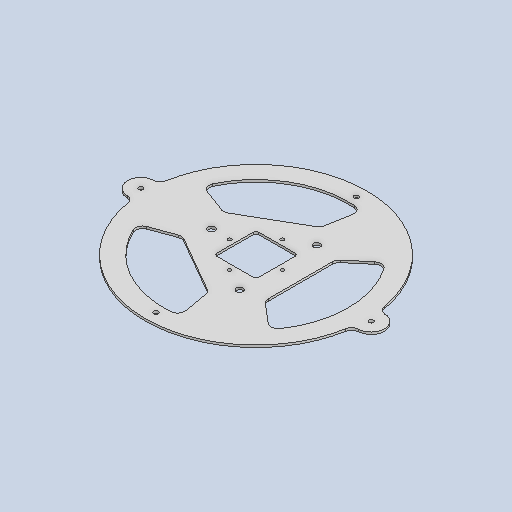
# Autodesk Inventor part: Part1
Saved by Autodesk Inventor 2025.1 (Build 291241020, 241B)
## iProperties
Created: 2024-10-16
Part Number: Part1
Material: Generic
Document SubType Name: Modeling
Designer: jdl5984
Density: 1 g/cm^3
Appearance: Default
Author: jdl5984
Autodesk Inventor part; units mm, degrees
ref_plane "YZ Plane" through (0, 0, 0) normal (1, 0, 0) x (0, 1, 0)
ref_plane "XZ Plane" through (0, 0, 0) normal (0, 1, 0) x (-1, 0, 0)
ref_plane "XY Plane" through (0, 0, 0) normal (0, 0, 1) x (1, 0, 0)
sketch "Sketch1" plane through (0, 0, 0) normal (0, 1, 0) x (-1, 0, 0)
  circle A0 centre (0, 0) radius 158.75
  line L0 (26.05, 30.05) -> (-26.05, 30.05)
  line L1 (-30.05, 26.05) -> (-30.05, -26.05)
  line L2 (-26.05, -30.05) -> (26.05, -30.05)
  line L3 (30.05, -26.05) -> (30.05, 26.05)
  arc A1 (30.05, 26.05) -> (26.05, 30.05) centre (26.05, 26.05) ccw
  arc A2 (26.05, -30.05) -> (30.05, -26.05) centre (26.05, -26.05) ccw
  arc A3 (-30.05, -26.05) -> (-26.05, -30.05) centre (-26.05, -26.05) ccw
  arc A4 (-26.05, 30.05) -> (-30.05, 26.05) centre (-26.05, 26.05) ccw
  circle A5 centre (38, 0) radius 2.5527
  circle A6 centre (0, -38) radius 2.5527
  circle A7 centre (-38, 0) radius 2.5527
  circle A8 centre (0, 38) radius 2.5527
  circle A9 centre (63.9092, 0) radius 4.7625
  circle A10 centre (-31.9546, -55.3454) radius 4.7625
  circle A11 centre (0, 0) radius 63.9092 construction
  circle A12 centre (0, 143.6497) radius 3.2067
  circle A13 centre (0, -143.6497) radius 3.2067
  line L4 (157.6029, 19.05) -> (165.227, 19.05)
  line L5 (165.227, 19.05) -> (165.227, -19.05) construction
  line L6 (165.227, -19.05) -> (157.6029, -19.05)
  line L7 (157.6029, -17.4578) -> (157.6029, 19.05) construction
  arc A14 (165.227, -19.05) -> (165.227, 19.05) centre (165.227, 0) ccw
  circle A15 centre (165.227, 0) radius 3.2067
  line L8 (0, -158.75) -> (0, 158.75) construction
  line L9 (-157.6029, 19.05) -> (-165.227, 19.05)
  line L10 (-165.227, -19.05) -> (-157.6029, -19.05)
  arc A16 (-165.227, 19.05) -> (-165.227, -19.05) centre (-165.227, 0) ccw
  circle A17 centre (-165.227, 0) radius 3.2067
  circle A18 centre (-31.9533, 55.3478) radius 4.7625
  point P0 (30.05, 30.05)
  point P1 (-30.05, 30.05)
  point P2 (30.05, -30.05)
  dimension "d0" = 317.5
  dimension "d1" = 30.05
  dimension "d2" = 60.1
  dimension "d3" = 60.1
  dimension "d4" = 30.05
  dimension "d5" = 4
  dimension "d6" = 4
  dimension "d7" = 5.1054
  dimension "d8" = 5.1054
  dimension "d9" = 5.1054
  dimension "d10" = 5.1054
  dimension "d11" = 76
  dimension "d12" = 38
  dimension "d13" = 76
  dimension "d14" = 38
  dimension "d15" = 9.525
  dimension "d17" = 110.6932
  dimension "d20" = 9.525
  dimension "d24" = 6.4135
  dimension "d25" = 6.4135
  dimension "d26" = 287.2994
  dimension "d27" = 143.6497
  dimension "d30" = 38.1
  dimension "d31" = 6.4135
  dimension "d33" = 330.454
  dimension "d38" = 110.6932
  dimension "d39" = 110.6932
  dimension "d41" = 127.8184
  constraints: 22 end point, 20 point on circle, 19 centre point, 8 tangent, 6 point on line, 6 symmetric about line, 4 coincident, 4 horizontal alignment, 4 parallel, 4 vertical alignment, 3 equal radius, 2 horizontal, 2 perpendicular, 1 midpoint, 1 vertical, 2 other
  measures "d0" diameter of A0
  measures "d1" distance from line of point (0, 0) L3
  measures "d2" distance of point (30.05, 30.05) point (-30.05, 30.05)
  measures "d3" distance of point (30.05, -30.05) point (30.05, 30.05)
  measures "d4" distance from line of point (0, 0) L2
  measures "d5" radius of A1
  measures "d6" radius of A2
  measures "d7" diameter of A5
  measures "d8" diameter of A6
  measures "d9" diameter of A7
  measures "d10" diameter of A8
  measures "d11" distance of A7.centre A5.centre
  measures "d12" distance of point (0, 0) A7.centre
  measures "d13" distance of A8.centre A6.centre
  measures "d14" distance of point (0, 0) A6.centre
  measures "d15" diameter of A9
  measures "d17" distance of A10.centre A9.centre
  measures "d20" diameter of A10
  measures "d24" diameter of A13
  measures "d25" diameter of A12
  measures "d26" distance of A13.centre A12.centre
  measures "d27" distance of A12.centre point (0, 0)
  measures "d30" distance of L4.start L6.end
  measures "d31" diameter of A15
  measures "d33" distance of A17.centre A14.centre
  measures "d38" distance of A18.centre A10.centre
  measures "d39" distance of A9.centre A18.centre
  measures "d41" diameter of A11
extrude "Extrusion1" add sketch "Sketch1" along normal blind 3.175
fillet "Fillet1" radius 10.16 4 edges at (-157.6029, 1.5875, 19.05) (-157.6029, 1.5875, -19.05) (157.6029, 1.5875, -19.05) (157.6029, 1.5875, 19.05)
sketch "Sketch2" plane through (0, 3.175, 0) normal (0, 1, 0) x (1, 0, 0)
  line L0 (63.5, 50.8) -> (102.4151, 83.4536)
  line L1 (63.5, 50.8) -> (63.5, -50.8)
  line L2 (63.5, -50.8) -> (102.4151, -83.4536)
  arc A0 (102.4151, -83.4536) -> (102.4151, 83.4536) centre (0, 0) ccw
  line L3 (-75.7441, 29.5926) -> (-123.4805, 46.9672)
  line L4 (12.2441, 80.3926) -> (21.0654, 130.4208)
  line L5 (-75.7441, 29.5926) -> (12.2441, 80.3926)
  arc A1 (21.0654, 130.4208) -> (-123.4805, 46.9672) centre (0, 0) ccw
  line L6 (12.2441, -80.3926) -> (21.0654, -130.4208)
  line L7 (-75.7441, -29.5926) -> (-123.4805, -46.9672)
  line L8 (12.2441, -80.3926) -> (-75.7441, -29.5926)
  arc A2 (-123.4805, -46.9672) -> (21.0654, -130.4208) centre (0, 0) ccw
  point P0 (0, 0)
  dimension "d42" = 101.6
  dimension "d43" = 50.8
  dimension "d44" = 130
  dimension "d45" = 130
  dimension "d46" = 50.8
  dimension "d47" = 50.8
  dimension "d48" = 63.5
  dimension "d49" = 0
  dimension "d52" = 360
  constraints: 18 end point, 6 point on circle, 3 centre point, 1 vertical, 28 other
  measures "d42" distance of L0.start L1.end
  measures "d43" vertical distance of point (0, 0) L0.start
  measures "d44" angle of L1 L2
  measures "d45" angle of L1 L0
  measures "d46" distance of L0.start L0.end
  measures "d47" distance of L1.end L2.end
  measures "d48" distance from line of point (0, 0) L1
  measures "d49" distance of point (0, 0) A0.centre
extrude "Extrusion2" cut sketch "Sketch2" against normal blind 6.35
fillet "Fillet2" radius 10.16 6 edges at (-123.4805, 1.5875, 46.9672) (21.0654, 1.5875, -130.4208) (102.4151, 1.5875, -83.4536) (21.0654, 1.5875, 130.4208) (102.4151, 1.5875, 83.4536) (-123.4805, 1.5875, -46.9672)
fillet "Fillet3" radius 10.16 6 edges at (-75.7441, 1.5875, -29.5926) (63.5, 1.5875, -50.8) (12.2441, 1.5875, 80.3926) (-75.7441, 1.5875, 29.5926) (63.5, 1.5875, 50.8) (12.2441, 1.5875, -80.3926)
sketch "Sketch3" plane through (0, 3.175, 0) normal (0, 1, 0) x (1, 0, 0)
  arc A0 (156.3619, 27.432) -> (-156.3619, 27.432) centre (0, 0) ccw projected
  line L0 (82.2664, 135.7711) -> (76.6274, 126.5262)
  line L1 (71.6492, 125.9572) -> (67.3261, 130.3685)
  line L2 (62.348, 129.7996) -> (52.2012, 113.1643)
  line L3 (54.9118, 108.336) -> (59.8766, 108.336)
  line L4 (62.5872, 103.5077) -> (59.6212, 98.6449)
  line L5 (62.1502, 93.8218) -> (68.5548, 93.4551)
  line L6 (70.903, 88.3667) -> (56.7738, 69.7364)
  line L7 (51.3067, 70.4499) -> (48.2668, 77.8597)
  line L8 (43.6958, 79.3771) -> (21.3897, 65.9934)
  line L9 (19.9367, 64.015) -> (15.5672, 45.89)
  line L10 (18.312, 41.9894) -> (42.8589, 39.3314)
  line L11 (45.5063, 35.1047) -> (41.1925, 23.0559)
  line L12 (39.4084, 21.1887) -> (30.05, 17.3494)
  line L13 (30.05, 26.05) -> (30.05, -26.05) projected
  arc A1 (71.6492, 125.9572) -> (76.6274, 126.5262) centre (73.9169, 128.1795) ccw
  arc A2 (67.3261, 130.3685) -> (62.348, 129.7996) centre (65.0585, 128.1462) ccw
  arc A3 (52.2012, 113.1643) -> (54.9118, 108.336) centre (54.9118, 111.511) ccw
  arc A4 (70.903, 88.3667) -> (68.5548, 93.4551) centre (68.3733, 90.2853) ccw
  arc A5 (62.5872, 103.5077) -> (59.8766, 108.336) centre (59.8766, 105.161) ccw
  arc A6 (51.3067, 70.4499) -> (56.7738, 69.7364) centre (54.2441, 71.655) ccw
  arc A7 (48.2668, 77.8597) -> (43.6958, 79.3771) centre (45.3294, 76.6546) ccw
  arc A8 (21.3897, 65.9934) -> (19.9367, 64.015) centre (23.0232, 63.2709) ccw
  arc A9 (15.5672, 45.89) -> (18.312, 41.9894) centre (18.6538, 45.1459) ccw
  arc A10 (45.5063, 35.1047) -> (42.8589, 39.3314) centre (42.5171, 36.1749) ccw
  arc A11 (39.4084, 21.1887) -> (41.1925, 23.0559) centre (38.2034, 24.1261) ccw
  arc A12 (59.6212, 98.6449) -> (62.1502, 93.8218) centre (62.3317, 96.9916) ccw
  line L14 (-157.7126, 3.3351) -> (-147.8886, 3.0982)
  line L15 (-144.9068, -0.9286) -> (-146.5655, -6.8781)
  line L16 (-143.5837, -10.9049) -> (-124.1038, -11.3746)
  line L17 (-121.2776, -6.613) -> (-123.76, -2.3133)
  arc A13 (-120.9339, 2.4483) -> (-123.76, -2.3133) centre (-121.0104, -0.7258) ccw
  arc A14 (-124.1038, -11.3746) -> (-121.2776, -6.613) centre (-124.0272, -8.2005) ccw
  arc A15 (-144.9068, -0.9286) -> (-147.8886, 3.0982) centre (-147.9651, -0.0759) ccw
  arc A16 (-146.5655, -6.8781) -> (-143.5837, -10.9049) centre (-143.5072, -7.7308) ccw
  line L18 (-120.9339, 2.4483) -> (-115.2396, 2.311)
  line L19 (-112.3272, 6.9128) -> (-115.2119, 12.6427)
  line L20 (-111.9793, 17.2205) -> (-88.7805, 14.2994)
  line L21 (-86.6648, 9.2079) -> (-91.5618, 2.8704)
  arc A17 (-111.9793, 17.2205) -> (-115.2119, 12.6427) centre (-112.376, 14.0704) ccw
  arc A18 (-115.2396, 2.311) -> (-112.3272, 6.9128) centre (-115.1631, 5.4851) ccw
  arc A19 (-91.5618, 2.8704) -> (-90.5905, -1.8469) centre (-89.0495, 0.9291) ccw
  arc A20 (-86.6648, 9.2079) -> (-88.7805, 14.2994) centre (-89.1771, 11.1492) ccw
  line L22 (-90.5905, -1.8469) -> (-67.8469, -14.4727)
  line L23 (-65.4069, -14.7418) -> (-47.5255, -9.4634)
  line L24 (-45.5199, -5.136) -> (-55.4915, 17.4512)
  line L25 (-53.1547, 21.8573) -> (-40.5633, 24.1458)
  line L26 (-38.0542, 23.5343) -> (-30.05, 17.3494)
  arc A21 (-67.8469, -14.4727) -> (-65.4069, -14.7418) centre (-66.3058, -11.6967) ccw
  arc A22 (-53.1547, 21.8573) -> (-55.4915, 17.4512) centre (-52.5869, 18.7334) ccw
  arc A23 (-47.5255, -9.4634) -> (-45.5199, -5.136) centre (-48.4244, -6.4183) ccw
  arc A24 (-38.0542, 23.5343) -> (-40.5633, 24.1458) centre (-39.9955, 21.022) ccw
  line L27 (76.448, -139.1304) -> (71.2612, -129.6244)
  line L28 (73.2575, -125.0287) -> (79.2394, -123.4904)
  line L29 (81.2357, -118.8947) -> (71.9026, -101.7897)
  line L30 (66.3658, -101.723) -> (63.8834, -106.0227)
  arc A25 (58.3467, -105.9559) -> (63.8834, -106.0227) centre (61.1338, -104.4352) ccw
  arc A26 (71.9026, -101.7897) -> (66.3658, -101.723) centre (69.1155, -103.3105) ccw
  arc A27 (73.2575, -125.0287) -> (71.2612, -129.6244) centre (74.0483, -128.1036) ccw
  arc A28 (79.2394, -123.4904) -> (81.2357, -118.8947) centre (78.4486, -120.4155) ccw
  line L31 (58.3467, -105.9559) -> (55.6184, -100.9559)
  line L32 (50.177, -100.7346) -> (46.6571, -106.0977)
  line L33 (41.0763, -105.5872) -> (32.0066, -84.0358)
  line L34 (35.3581, -79.6578) -> (43.2951, -80.7301)
  arc A29 (41.0763, -105.5872) -> (46.6571, -106.0977) centre (44.0027, -104.3556) ccw
  arc A30 (55.6184, -100.9559) -> (50.177, -100.7346) centre (52.8313, -102.4767) ccw
  arc A31 (43.2951, -80.7301) -> (46.8947, -77.5303) centre (43.7201, -77.5837) ccw
  arc A32 (35.3581, -79.6578) -> (32.0066, -84.0358) centre (34.933, -82.8043) ccw
  line L35 (46.8947, -77.5303) -> (46.4571, -51.5208)
  line L36 (45.4703, -49.2732) -> (31.9583, -36.4266)
  line L37 (27.2079, -36.8534) -> (12.6326, -56.7826)
  line L38 (7.6484, -56.9619) -> (-0.6292, -47.2018)
  line L39 (-1.3542, -44.7231) -> (0, -34.6988)
  arc A33 (46.4571, -51.5208) -> (45.4703, -49.2732) centre (43.2826, -51.5742) ccw
  arc A34 (7.6484, -56.9619) -> (12.6326, -56.7826) centre (10.0698, -54.9083) ccw
  arc A35 (31.9583, -36.4266) -> (27.2079, -36.8534) centre (29.7706, -38.7277) ccw
  arc A36 (-1.3542, -44.7231) -> (-0.6292, -47.2018) centre (1.7922, -45.1481) ccw
  line L40 (-30.05, -26.05) -> (-30.05, 26.05) projected
  line L41 (0, -34.6988) -> (0.628, -30.05)
  line L42 (26.05, -30.05) -> (-26.05, -30.05) projected
  line L43 (-159.5209, 3.9541) -> (-175.7168, 15.9018)
  arc A37 (-165.9718, 19.0354) -> (-165.9718, -19.0354) centre (-165.227, 0) ccw projected
  arc A38 (-159.5209, 3.9541) -> (-157.7126, 3.3351) centre (-157.6361, 6.5092) ccw
  point P0 (65.5323, 108.336)
  point P1 (56.8639, 94.1245)
  point P2 (-158.7145, 3.3592)
  point P3 (-126.5879, 2.5846)
  point P4 (-109.9462, 2.1833)
  point P5 (61.0556, -110.9206)
  point P6 (53.0823, -96.3078)
  dimension "d58" = 3.175
  dimension "d61" = 360
  dimension "d63" = 3.175
  constraints: 82 end point, 76 point on circle, 37 centre point, 26 tangent, 23 point on line, 11 equal radius, 4 coincident, 1 collinear, 1 horizontal, 1 parallel, 1 perpendicular, 196 other
  measures "d58" radius of A1
  measures "d63" radius of A38
split "Split5" [suppressed]
split "Split8" [suppressed]
split "Split9" [suppressed]
combine "Combine1" [suppressed]
feature "Move Body1" [suppressed]
feature "Move Body2" [suppressed]
feature "Move Body3" [suppressed]
feature "Move Body4" [suppressed]
feature "Move Body5" [suppressed]
equation "\"d24\" = d25"
equation "\"d25\" = d31"
equation "\"d38\" = d17"
equation "\"d39\" = d17"
body "Solid1"
body "Solid18"
body "Solid19"
body "Solid22"
body "Solid23"
body "Solid24"
body "Solid25"
